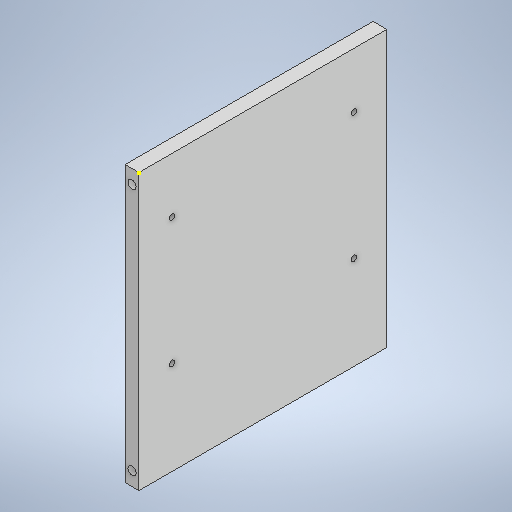
# Autodesk Inventor part: Atras
Saved by Autodesk Inventor 2025.2 (Build 292293000, 293)
## iProperties
Created: 2025-01-27
Part Number: Atras
Material: Genérico
Document SubType Name: Modeling
Designer: alex
Density: 1 g/cm^3
Appearance: Valor por defecto
Author: alex
Autodesk Inventor part; units mm, degrees
ref_plane "YZ Plane" through (0, 0, 0) normal (1, 0, 0) x (0, 1, 0)
ref_plane "XZ Plane" through (0, 0, 0) normal (0, 1, 0) x (-1, 0, 0)
ref_plane "XY Plane" through (0, 0, 0) normal (0, 0, 1) x (1, 0, 0)
sketch "Boceto1" plane through (0, 0, 0) normal (1, 0, 0) x (0, 1, 0)
  line L0 (0, 0) -> (-100, 0)
  line L1 (-100, 0) -> (-100, -90)
  line L2 (-100, -90) -> (0, -90)
  line L3 (0, -90) -> (0, 0)
  dimension "d0" = 90
  dimension "d1" = 100
  constraints: 8 end point, 2 parallel, 1 horizontal, 1 perpendicular
  measures "d0" distance between parallel lines of L0 L2
  measures "d1" distance between parallel lines of L1 L3
extrude "Extrusión1" add sketch "Boceto1" along normal blind 5
sketch "Boceto2" plane through (0, -100, 0) normal (0, 0, 1) x (1, 0, 0)
  line L0 (20, -20) -> (0, 0)
  line L1 (20, -20) -> (20, -15)
  line L2 (20, -15) -> (5, 0)
  line L3 (0, 0) -> (0, 100) projected
  line L4 (0, 0) -> (5, 0)
  dimension "d6" = 5
  constraints: 8 end point
  measures "d6" distance of L0.start L1.end
extrude "Extrusión2" add sketch "Boceto2" against normal blind 90
sketch "Boceto3" plane through (5, 0, -90) normal (0, 0, -1) x (-1, 0, 0)
  circle A0 centre (2.5, -5) radius 1.5
  circle A1 centre (2.5, -95) radius 1.5
  line L0 (5, -100) -> (5, 0) projected
  line L1 (5, 0) -> (0, 0) projected
  line L2 (0, -100) -> (0, 0) projected
  dimension "d9" = 3
  dimension "d10" = 3
  dimension "d11" = 2.5
  dimension "d12" = 5
  dimension "d13" = 5
  dimension "d14" = 2.5
  constraints: 2 centre point
  measures "d9" diameter of A0
  measures "d10" diameter of A1
  measures "d11" distance from line of L0 A1.centre
  measures "d12" vertical distance of L0.start A1.centre
  measures "d13" distance from line of L1 A0.centre
  measures "d14" distance from line of L2 A0.centre
extrude "Extrusión3" cut sketch "Boceto3" against normal blind 3
sketch "Boceto4" plane through (0, 0, 0) normal (0, 0, 1) x (1, 0, 0)
  circle A0 centre (2.5, -5) radius 1.5 projected
  circle A1 centre (2.5, -5) radius 1.5
  circle A2 centre (2.5, -95) radius 1.5 projected
  circle A3 centre (2.5, -95) radius 1.5
  point P0 (0, 0)
  constraints: 2 centre point, 2 coincident
extrude "Extrusión4" cut sketch "Boceto4" against normal blind 3
sketch "Boceto5" plane through (0, 0, 0) normal (0, 0, 1) x (1, 0, 0)
  line L0 (0, 0) -> (0, -100) projected
  line L1 (20, -115) -> (5, -100) projected
  line L2 (0, -100) -> (5, -100)
  line L3 (5, -100) -> (2.5, -102.5)
  line L4 (0, -100) -> (20, -120) projected
  constraints: 4 end point, 1 horizontal, 1 point on line
extrude "Extrusión5" cut sketch "Boceto5" against normal blind 3000
sketch "Boceto6" plane through (5, 0, 0) normal (1, 0, 0) x (0, 0, -1)
  point P0 (0, 0)
sketch "Boceto7" plane through (20, -120, 0) normal (0, 0, 1) x (1, 0, 0)
  line L0 (-17.5, 17.5) -> (0, 0) projected
  line L1 (0, 5) -> (-15, 20) projected
  line L2 (-17.5, 17.5) -> (-15, 20)
  line L3 (0, 0) -> (0, 5) projected
  line L4 (-15, 20) -> (0, 5)
  line L5 (0, 5) -> (0, 0)
  line L6 (0, 0) -> (-17.5, 17.5)
  point P0 (-20, 120)
  constraints: 8 end point, 2 perpendicular, 1 parallel, 1 vertical
extrude "Extrusión6" cut sketch "Boceto7" against normal blind 3000
sketch "Boceto8" plane through (5, 0, 0) normal (1, 0, 0) x (0, 0, -1)
  circle A0 centre (12, -20) radius 1
  line L0 (0, 0) -> (0, -100) projected
  line L1 (90, 0) -> (0, 0) projected
  circle A1 centre (78, -20) radius 1
  circle A2 centre (12, -66) radius 1
  circle A3 centre (78, -66) radius 1
  dimension "d23" = 2
  dimension "d24" = 12
  dimension "d25" = 20
  dimension "d26" = 2
  dimension "d27" = 66
  dimension "d28" = 20
  dimension "d29" = 2
  dimension "d30" = 2
  dimension "d31" = 46
  dimension "d32" = 46
  dimension "d33" = 66
  constraints: 4 centre point
  measures "d23" diameter of A0
  measures "d24" distance from line of L0 A0.centre
  measures "d25" distance from line of L1 A0.centre
  measures "d26" diameter of A1
  measures "d27" distance of A1.centre A0.centre
  measures "d28" distance from line of L1 A1.centre
  measures "d29" diameter of A2
  measures "d30" diameter of A3
  measures "d31" distance of A0.centre A2.centre
  measures "d32" distance of A1.centre A3.centre
  measures "d33" distance of A3.centre A2.centre
extrude "Extrusión7" cut sketch "Boceto8" against normal blind 5
